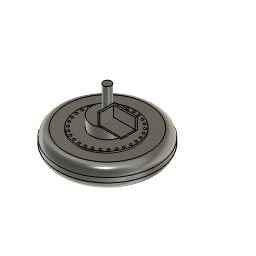
frame v2 (Autodesk Fusion 360 design; units mm, degrees)
Autodesk Fusion 360 part; units mm, degrees
sketch "Sketch1" plane through (0, 0, 0) normal (0, 0, 1) x (1, 0, 0)
  circle A0 centre (0, 0) radius 125
  dimension "d2" = 250
  constraint coincident A0.centre origin
  measures "d2" diameter of A0
extrude "Extrude1" add sketch "Sketch1" along normal blind 60 makes body 1
sketch "Sketch2" plane through (0, 0, 60) normal (0, 0, 1) x (-1, 0, 0)
  circle A0 centre (0, 0) radius 125
  circle A1 centre (0, 0) radius 40
  dimension "d5" = 80
  constraint coincident A0.centre A1.centre
  measures "d5" diameter of A1
extrude "Extrude2" add sketch "Sketch2" along normal blind 30 contours A1 bodies 1
sketch "Sketch3" plane through (0, 0, 0) normal (0, 0, 1) x (1, 0, 0)
  circle A0 centre (0, 0) radius 125.1705
  constraint coincident A0.centre origin
extrude "Extrude3" cut sketch "Sketch3" along normal blind 10 bodies 1
extrude "Extrude4" add 1 faces at (-13.1545, 45.4909, 10) along direction (0, 0, -1) blind 1 on bodies 1 bodies 1
extrude "Extrude5" add 1 faces at (96.0524, -8.1973, 60) along direction (0, 0, 1) blind 1 on bodies 1 bodies 1
fillet "Fillet1" radius 20 1 edges at (-116.5409, -45.2019, 61) on bodies 1
fillet "Fillet2" radius 20 1 edges at (-116.5409, 45.2019, 9) on bodies 1
sketch "Sketch4" plane through (0, 0, 90) normal (0, 0, 1) x (-1, 0, 0)
  circle A0 centre (0, 0) radius 40
  circle A1 centre (-230, 0) radius 37.5
  dimension "d18" = 75
  measures "d18" diameter of A1
extrude "Extrude6" add sketch "Sketch4" along normal blind 2 separate body contours A1 makes body 2
sketch "Sketch5" plane through (0, 0, 92) normal (0, 0, 1) x (-1, 0, 0)
  circle A0 centre (-230, 0) radius 37.5
hole "Hole1" at (229.9535, -34.6096, 92) direction (0, 0, -1) diameter 3 depth 25 tip angle 118 bodies 2
pattern_circular "C-Pattern2" count 30 over 360 about axis through (230, 0, 17) along (0, 0, 1) of "Hole1"
scale "Scale2" factor 2 about (195.4183, -2.0797, 90) bodies 2
hole "Hole32" at (265.0338, 3.9, 94) direction (0, 0, -1) diameter 80 depth 25 tip angle 118 bodies 2
move_body "Move1" bodies 2 to x (1, 0, 0) y (0, 1, 0) z (0, 0, 1) at (-265, -4.0665, 0)
move_body "Move2" bodies 2 to x (1, 0, 0) y (0, 1, 0) z (0, 0, 1) at (0, 0, -30)
hole "Hole33" at (0, 0, 92) direction (0, 0, -1) diameter 20 end through all bodies 1
sketch "Sketch6" plane through (0, 0, 0) normal (1, 0, 0) x (0, 1, 0)
sketch "Sketch7" plane through (0, 0, 0) normal (0, 0, 1) x (1, 0, 0)
  line L0 (95.9005, -150) -> (155.9005, -150)
  line L1 (155.9005, -150) -> (155.9005, -190)
  line L2 (155.9005, -190) -> (95.9005, -190)
  line L3 (95.9005, -190) -> (95.9005, -150)
  line L4 (95.9005, -150) -> (100.9005, -150)
  line L5 (100.9005, -155) -> (100.9005, -190)
  line L6 (100.9005, -190) -> (95.9005, -190)
  line L7 (95.9005, -190) -> (95.9005, -150)
  line L8 (95.9005, -150) -> (155.9005, -150)
  line L9 (155.9005, -150) -> (155.9005, -155)
  line L10 (155.9005, -155) -> (100.9005, -155)
  line L11 (95.9005, -155) -> (95.9005, -150)
  constraint horizontal L0
  constraint vertical L1
  constraint horizontal L2
  constraint vertical L3
  constraint vertical L5
  constraint horizontal L6
  constraint vertical L7
  constraint horizontal L8
  constraint vertical L9
  constraint horizontal L10
extrude "Extrude7" add sketch "Sketch7" along normal blind 30 separate body contours L0 L1 L2 L3 L4 L5 L6 L7 L8 L9 L10 L11 makes body 3
sketch "Sketch8" plane through (0, 0, 0) normal (0, 0, 1) x (1, 0, 0)
move_body "Move3" bodies 3 to x (1, 0, 0) y (0, 1, 0) z (0, 0, 1) at (-85, 155, 90)
sketch "Sketch10" plane through (0, 0, 0) normal (1, 0, 0) x (0, 1, 0)
sketch "Sketch11" plane through (0, 0, 0) normal (0, 0, 1) x (1, 0, 0)
  line L0 (-270, 0) -> (-200.5177, 0)
  line L1 (-200.5177, 0) -> (-200.5177, -38.0447)
  line L2 (-200.5177, -38.0447) -> (-270, -38.0447)
  line L3 (-270, -38.0447) -> (-270, 0)
  constraint horizontal L0
  constraint vertical L1
  constraint horizontal L2
  constraint vertical L3
extrude "Extrude8" add sketch "Sketch11" along normal blind 5 separate body makes body 4
move_face "MoveFace2" by (13.5256, 0, -1.5532) 1 faces at (-246.8392, -25.3631, 5) on bodies 4
move_body "Move4" bodies 4 to x (1, 0, 0) y (0, 1, 0) z (0, 0, 1) at (280, 0, 90)
extrude "Extrude9" cut 1 faces at (79.4823, -12.6816, 92.2979) along direction (-1, 0, 0) blind 8.5 on bodies 4 bodies 4
extrude "Extrude10" cut 1 faces at (50.6549, -38.0447, 91.1489) along direction (0, 1, 0) blind 3 on bodies 4 bodies 4
extrude "Extrude11" cut 1 faces at (10, -23.3631, 91.1489) along direction (1, 0, 0) blind 1 on bodies 4 bodies 3 4
sketch "Sketch12" plane through (0, 0, 0) normal (1, 0, 0) x (0, 1, 0)
sketch "Sketch13" plane through (0, 0, 90) normal (0, 0, 1) x (-1, 0, 0)
  circle A0 centre (0, 0) radius 10
  circle A1 centre (0, 0) radius 40
  circle A2 centre (0, 0) radius 10
  constraint coincident A0.centre A1.centre
extrude "Extrude12" add sketch "Sketch13" along normal mid plane 140 contours A0 A2 bodies 1
